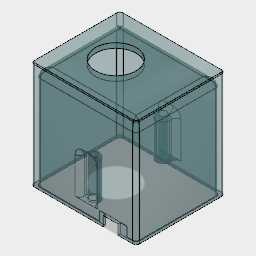
Save Button (Autodesk Fusion 360 design; units mm, degrees)
Autodesk Fusion 360 part; units mm, degrees
sketch "Sketch1" plane through (0, 0, 0) normal (0, 1, 0) x (1, 0, 0)
  line L0 (12, -4.9972) -> (73, -4.9972)
  line L1 (75, -6.9972) -> (75, -57.9994)
  line L2 (73, -59.9994) -> (12, -59.9994)
  line L3 (10, -57.9994) -> (10, -6.9972)
  arc A0 (12, -4.9972) -> (10, -6.9972) centre (12, -6.9972) ccw
  arc A1 (75, -6.9972) -> (73, -4.9972) centre (73, -6.9972) ccw
  arc A2 (73, -59.9994) -> (75, -57.9994) centre (73, -57.9994) ccw
  arc A3 (10, -57.9994) -> (12, -59.9994) centre (12, -57.9994) ccw
  line L4 (71.0012, -58) -> (14.0012, -58)
  line L5 (12.0012, -56) -> (12.0012, -9)
  line L6 (14.0012, -7) -> (71.0012, -7)
  line L7 (73.0012, -9) -> (73.0012, -56)
  arc A4 (14.0012, -7) -> (12.0012, -9) centre (14.0012, -9) ccw
  arc A5 (73.0012, -9) -> (71.0012, -7) centre (71.0012, -9) ccw
  arc A6 (71.0012, -58) -> (73.0012, -56) centre (71.0012, -56) ccw
  arc A7 (12.0012, -56) -> (14.0012, -58) centre (14.0012, -56) ccw
  line L8 (10, -32.4983) -> (75, -32.4983) construction
  line L9 (35, -4.9972) -> (35, -59.9994) construction
  circle A8 centre (35, -32.4983) radius 12.5
  line L10 (50, -4.9972) -> (50, -59.9994) construction
  line L11 (50, -58.4994) -> (85, -58.4994) construction
  line L12 (50, -58.4994) -> (68.5, -58.4994)
  line L13 (68.5, -58.4994) -> (68.5, -21.7494)
  line L14 (68.5, -21.7494) -> (50, -21.7494)
  line L15 (50, -21.7494) -> (50, -58.4994)
  line L16 (59.25, -21.7494) -> (59.25, -69.0332) construction
  line L17 (54.75, -58.4994) -> (63.75, -58.4994)
  line L18 (63.75, -58.4994) -> (63.75, -61.4994)
  line L19 (63.75, -61.4994) -> (54.75, -61.4994)
  line L20 (54.75, -61.4994) -> (54.75, -58.4994)
  line L21 (67.7, -21.7494) -> (67.7, -58.4994)
  line L22 (50.8, -21.7494) -> (50.8, -58.4994)
  line L23 (42.5012, -7) -> (42.5012, -58) construction
  circle A9 centre (42.5012, -53.9885) radius 2.25
  circle A10 centre (42.5012, -53.9885) radius 4
  circle A11 centre (42.5012, -53.9885) radius 1.6
  circle A12 centre (42.5012, -11.0081) radius 4
  circle A13 centre (42.5012, -11.0081) radius 2.25
  circle A14 centre (42.5012, -11.0081) radius 1.6
  line L24 (46.5012, -53.9885) -> (46.5012, -58.2)
  line L25 (38.5012, -53.9885) -> (38.5012, -58.2)
  line L26 (38.5012, -11.0081) -> (38.5012, -6.8)
  line L27 (46.5012, -11.0081) -> (46.5012, -6.8)
  circle A15 centre (42.5012, -11.0081) radius 3
  circle A16 centre (42.5012, -53.9885) radius 3
  arc A17 (73.2012, -9) -> (71.0012, -6.8) centre (71.0012, -9) ccw
  line L28 (14.0012, -6.8) -> (71.0012, -6.8)
  arc A18 (14.0012, -6.8) -> (11.8012, -9) centre (14.0012, -9) ccw
  line L29 (11.8012, -56) -> (11.8012, -9)
  arc A19 (11.8012, -56) -> (14.0012, -58.2) centre (14.0012, -56) ccw
  line L30 (71.0012, -58.2) -> (14.0012, -58.2)
  arc A20 (71.0012, -58.2) -> (73.2012, -56) centre (71.0012, -56) ccw
  line L31 (73.2012, -9) -> (73.2012, -56)
  dimension "d4" = 2
  dimension "d5" = 2
  dimension "d6" = 25
  dimension "d7" = 25
  dimension "d8" = 15
  dimension "d9" = 1.5
  dimension "d10" = 18.5
  dimension "d11" = 36.75
  dimension "d12" = 9
  dimension "d13" = 3
  dimension "d14" = 0.8
  dimension "d27" = 4.5
  dimension "d28" = 8
  dimension "d29" = 3.2
  dimension "d33" = 0.2
  dimension "d54" = 6
  constraint horizontal L0
  constraint vertical L1
  constraint horizontal L2
  constraint vertical L3
  constraint tangent L0 A0
  constraint tangent L3 A0
  constraint tangent L0 A1
  constraint tangent L1 A1
  constraint equal A0 A1
  constraint tangent L1 A2
  constraint tangent L2 A2
  constraint equal A0 A2
  constraint tangent L2 A3
  constraint tangent L3 A3
  constraint equal A0 A3
  constraint parallel L2 L4
  constraint parallel L3 L5
  constraint parallel L0 L6
  constraint parallel L1 L7
  constraint tangent L5 A4
  constraint tangent L6 A4
  constraint tangent L6 A5
  constraint tangent L7 A5
  constraint equal A4 A5
  constraint tangent L4 A6
  constraint tangent L7 A6
  constraint equal A4 A6
  constraint tangent L4 A7
  constraint tangent L5 A7
  constraint equal A4 A7
  constraint midpoint L3 origin
  constraint midpoint L1 origin
  constraint coincident L2
  constraint perpendicular L2 L9
  constraint midpoint L9 origin
  constraint perpendicular L2 L10
  constraint coincident L10
  constraint perpendicular L10 L11
  constraint horizontal L12
  constraint vertical L13
  constraint horizontal L14
  constraint vertical L15
  constraint midpoint L14 origin
  constraint vertical L16
  constraint horizontal L17
  constraint vertical L18
  constraint horizontal L19
  constraint vertical L20
  constraint coincident L11
  constraint midpoint L19 origin
  constraint coincident L16 origin
  constraint coincident L14 origin
  constraint perpendicular L14 L21
  constraint coincident L12
  constraint midpoint L6
  constraint perpendicular L6 L23
  constraint coincident L23
  constraint concentric A9 A10
  constraint concentric A9 A11
  constraint coincident A10 origin
  constraint coincident L30
  constraint tangent A10 L25
  constraint tangent A10 L24
  constraint perpendicular L24 L30
  constraint perpendicular L25 L30
  constraint coincident L28
  constraint perpendicular L26 L28
  constraint perpendicular L27 L28
  constraint concentric A14 A15
  measures "d4" radius of A0
  measures "d5" radius of A4
  measures "d6" distance of L3 L9
  measures "d7" diameter of A8
  measures "d8" distance of L9 L10
  measures "d9" distance of L2 L11
  measures "d11" distance of origin
  measures "d13" distance of origin
  measures "d14" distance of L13 L21
  measures "d27" diameter of A9
  measures "d28" diameter of A10
  measures "d29" diameter of A11
  measures "d54" diameter of A15
extrude "Extrude1" add sketch "Sketch1" along normal blind 1 contours L0 L1 L2 L3 A0 A1 A2 A3 L12 L13 L15 L18 L20 A17 L28 A18 L29 A19 L30 A20 L31 | L2 L12 L17 L18 L20 | L12 L17 L21 L22 L30 | L12 L15 L22 L30 | L12 L13 L21 L30 | L4 L15 L22 L30 | L4 L21 L22 L30 | L4 L13 L21 L30 | L4 L15 L24 L30 | L4 L14 L21 L22 | L4 L14 L15 L22 | L4 L6 L7 A5 A6 L13 L27 A17 L28 L30 A20 L31 | L4 L13 L14 L21 | L4 L5 L6 L7 A4 A5 A6 A7 L13 L14 L15 A10 A12 L24 L25 L26 L27 | L4 L24 L25 L30 | L4 A10 L24 L25 | L4 L5 L6 A4 A7 L25 L26 L28 A18 L29 A19 L30 | A10 | L6 L26 L27 L28 | L6 A12 L26 L27 | A12 | A8 | A9 | A11 | A13 | A14 | A15 | A16 makes body 1
extrude "Extrude2" add sketch "Sketch1" along normal blind 5 separate body contours L4 L5 L6 L7 A4 A5 A6 A7 L13 L14 L15 A10 A12 L24 L25 L26 L27 | L4 A10 L24 L25 | A10 | L6 A12 L26 L27 | A12 | A8 | A9 | A11 | A13 | A14 | A15 | A16 makes body 2
extrude "Extrude3" add sketch "Sketch1" along normal blind 2 contours L4 L14 L15 L22 | L4 L13 L14 L21 bodies 1 2
extrude "Extrude4" add sketch "Sketch1" along normal blind 5 and the other way blind -4 contours L4 L14 L15 L22 | L4 L13 L14 L21 bodies 1
fillet "Fillet1" radius 1 2 edges at (67.7, 4, 39.8747) (50.8, 4, 39.8747) on bodies 1
extrude "Extrude5" cut sketch "Sketch1" along normal up to surface (5 mm away) contours A11 | A14 bodies 1
extrude "Extrude6" cut sketch "Sketch1" along normal blind 3.1 contours A9 | A13 | A15 | A16 bodies 1
extrude "Extrude7" add sketch "Sketch1" along normal blind 63 separate body contours L0 L1 L2 L3 A0 A1 A2 A3 L12 L13 L15 L18 L20 A17 L28 A18 L29 A19 L30 A20 L31 | L2 L12 L17 L18 L20 | L12 L17 L21 L22 L30 | L12 L15 L22 L30 | L12 L13 L21 L30 makes body 3
extrude "Extrude8" add sketch "Sketch1" along normal blind 30 and the other way blind -6 contours L4 L24 L25 L30 | L4 A10 L24 L25 | A10 | L6 L26 L27 L28 | L6 A12 L26 L27 | A12 | A15 | A16 bodies 3
fillet "Fillet2" radius 1.75 6 edges at (46.5012, 30, 56.0943) (42.5012, 30, 49.9885) (38.5012, 30, 56.0943) (38.5012, 30, 8.9041) (42.5012, 30, 15.0081) (46.5012, 30, 8.9041) on bodies 3
extrude "Extrude9" add sketch "Sketch1" along normal blind 66 and the other way blind -63 contours L0 L1 L2 L3 A0 A1 A2 A3 L12 L13 L15 L18 L20 A17 L28 A18 L29 A19 L30 A20 L31 | L2 L12 L17 L18 L20 | L12 L17 L21 L22 L30 | L12 L15 L22 L30 | L12 L13 L21 L30 | L4 L15 L22 L30 | L4 L21 L22 L30 | L4 L13 L21 L30 | L4 L15 L24 L30 | L4 L14 L21 L22 | L4 L14 L15 L22 | L4 L6 L7 A5 A6 L13 L27 A17 L28 L30 A20 L31 | L4 L13 L14 L21 | L4 L5 L6 L7 A4 A5 A6 A7 L13 L14 L15 A10 A12 L24 L25 L26 L27 | L4 L24 L25 L30 | L4 A10 L24 L25 | L4 L5 L6 A4 A7 L25 L26 L28 A18 L29 A19 L30 | A10 | L6 L26 L27 L28 | L6 A12 L26 L27 | A12 | A9 | A11 | A13 | A14 | A15 | A16 bodies 3
fillet "Fillet3" radius 3 5 edges at (46.5012, 17.125, 58.2) (45.9886, 29.4874, 58.2) (42.5012, 30, 58.2) (39.0138, 29.4874, 58.2) (38.5012, 17.125, 58.2) on bodies 3
fillet "Fillet4" radius 0.5 8 edges at (75, 66, 32.4983) (74.4142, 66, 5.583) (42.5, 66, 4.9972) (10.5858, 66, 5.583) (10, 66, 32.4983) (10.5858, 66, 59.4136) (42.5, 66, 59.9994) (74.4142, 66, 59.4136) on bodies 3
fillet "Fillet10" radius 3 5 edges at (38.5012, 17.125, 6.8) (39.0138, 29.4874, 6.8) (42.5012, 30, 6.8) (45.9886, 29.4874, 6.8) (46.5012, 17.125, 6.8) on bodies 3
fillet "Fillet5" radius 0.25 8 edges at (42.5012, 0, 58.2) (12.4456, 0, 57.5556) (11.8012, 0, 32.5) (12.4456, 0, 7.4444) (42.5012, 0, 6.8) (72.5568, 0, 7.4444) (73.2012, 0, 32.5) (72.5568, 0, 57.5556) on bodies 3
fillet "Fillet6" radius 5 8 edges at (42.5012, 63, 58.2) (12.4456, 63, 57.5556) (11.8012, 63, 32.5) (12.4456, 63, 7.4444) (42.5012, 63, 6.8) (72.5568, 63, 7.4444) (73.2012, 63, 32.5) (72.5568, 63, 57.5556) on bodies 3
fillet "Fillet7" radius 0.25 8 edges at (10.5858, 0, 59.4136) (10, 0, 32.4983) (10.5858, 0, 5.583) (42.5, 0, 4.9972) (74.4142, 0, 5.583) (75, 0, 32.4983) (74.4142, 0, 59.4136) (42.5, 0, 59.9994) on bodies 1
fillet "Fillet8" radius 0.25 9 edges at (69.3506, 5, 58) (72.4154, 5, 57.4142) (73.0012, 5, 32.5) (72.4154, 5, 7.5858) (42.5012, 5, 7) (12.587, 5, 7.5858) (12.0012, 5, 32.5) (12.587, 5, 57.4142) (32.4006, 5, 58) on bodies 1
extrude "Extrude10" cut sketch "Sketch1" along normal blind 6 contours L2 L12 L17 L18 L20 | L2 L18 L19 L20 | L12 L17 L21 L22 L30 bodies 3
fillet "Fillet11" radius 0.5 2 edges at (40.4035, 6, 53.1749) (40.4035, 6, 10.1945) on bodies 3
hidden bodies 1
equation "d6 = 23 mm + 2 mm"
equation "d43 = 3 mm"
equation "d52 = d43"
named bodies: "Bottom Lid", "Switch Body"
